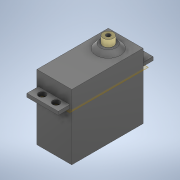
# Autodesk Inventor part: HX-15CS_15KGs_metal_gear_servo
Saved by Autodesk Inventor 2020 (Build 240168000, 168)
## iProperties
Created: 2019-12-03
Part Number: HX-15CS_15KGs_metal_gear_servo
Material: Generic
Document SubType Name: Modeling
Designer: maste
Density: 1 g/cm^3
Appearance: Smooth - Black
Author: maste
Autodesk Inventor part; units mm, degrees
ref_plane "YZ Plane" through (0, 0, 0) normal (1, 0, 0) x (0, 1, 0)
ref_plane "XY Plane" through (0, 0, 0) normal (0, 0, 1) x (1, 0, 0)
sketch "Sketch1" plane through (0, 0, 0) normal (0, 1, 0) x (-1, 0, 0)
  line L0 (20, 0) -> (0, 0)
  line L1 (0, 0) -> (0, -41)
  line L2 (0, -41) -> (20, -41)
  line L3 (20, -41) -> (20, 0)
  dimension "d0" = 20
  dimension "d1" = 41
  constraints: 8 end point, 2 parallel, 1 coincident, 1 horizontal, 1 perpendicular
  measures "d0" distance of L0.start L0.end
  measures "d1" distance of L0.end L1.end
extrude "Extrusion1" add sketch "Sketch1" along normal blind 37.5
sketch "Sketch2" plane through (0, 37.5, 0) normal (0, 1, 0) x (1, 0, 0)
  circle A0 centre (-10, 31) radius 3
  line L0 (-20, 41) -> (-20, 0) projected
  line L1 (0, 41) -> (-20, 41) projected
  point P0 (0, 0)
  dimension "d4" = 6
  dimension "d5" = 10
  dimension "d6" = 10
  constraints: 1 centre point
  measures "d4" diameter of A0
  measures "d5" distance from line of L0 A0.centre
  measures "d6" distance from line of L1 A0.centre
extrude "Extrusion2" add sketch "Sketch2" along normal blind 6.5
sketch "Sketch3" plane through (0, 37.5, 0) normal (0, 1, 0) x (1, 0, 0)
  circle A0 centre (-10, 31) radius 3 projected
  circle A1 centre (-10, 31) radius 7
  point P0 (0, 0)
  dimension "d9" = 14
  constraints: 1 centre point, 1 coincident
  measures "d9" diameter of A1
extrude "Extrusion3" add sketch "Sketch3" along normal blind 2.5
chamfer "Chamfer1" distance 2.5 angle 45 1 edges at (-17, 40, -31)
ref_plane "Work Plane1" through (0, 27.5, 0) normal (0, 1, 0) x (-1, 0, 0)
sketch "Sketch4" plane through (0, 27.5, 0) normal (0, 1, 0) x (-1, 0, 0)
  line L0 (19, -47.75) -> (1, -47.75)
  line L1 (1, -47.75) -> (1, 6.75)
  line L2 (1, 6.75) -> (19, 6.75)
  line L3 (19, 6.75) -> (19, -47.75)
  line L4 (0, 0) -> (0, -41) projected
  line L5 (0, -41) -> (20, -41) projected
  line L6 (14, -44) -> (6, -44) construction
  line L7 (6, -44) -> (6, 3) construction
  line L8 (6, 3) -> (14, 3) construction
  line L9 (14, 3) -> (14, -44) construction
  circle A0 centre (14, -44) radius 2
  circle A1 centre (6, -44) radius 2
  circle A2 centre (14, 3) radius 2
  circle A3 centre (6, 3) radius 2
  dimension "d16" = 54.5
  dimension "d17" = 18
  dimension "d18" = 1
  dimension "d19" = 6.75
  dimension "d20" = 47
  dimension "d21" = 8
  dimension "d22" = 5
  dimension "d23" = 3.75
  dimension "d24" = 4
  dimension "d25" = 4
  dimension "d26" = 4
  dimension "d27" = 4
  constraints: 16 end point, 4 centre point, 4 coincident, 4 parallel, 2 horizontal, 2 perpendicular
  measures "d16" distance of L0.end L1.end
  measures "d17" distance of L0.start L0.end
  measures "d18" distance between parallel lines of L4 L1
  measures "d19" distance between parallel lines of L5 L0
  measures "d20" distance of L6.end L7.end
  measures "d21" distance of L6.start L6.end
  measures "d22" distance between parallel lines of L3 L9
  measures "d23" distance between parallel lines of L2 L8
  measures "d24" diameter of A0
  measures "d25" diameter of A1
  measures "d26" diameter of A2
  measures "d27" diameter of A3
extrude "Extrusion4" add sketch "Sketch4" along normal blind 2
sketch "Sketch5" plane through (-10, 44, -31) normal (0, 1, 0) x (1, 0, 0)
  circle A0 centre (0, 0) radius 3 projected
  circle A1 centre (0, 0) radius 1.25
  point P0 (10, -31)
  dimension "d30" = 2.5
  constraints: 1 centre point, 1 coincident
  measures "d30" diameter of A1
extrude "Extrusion5" cut sketch "Sketch5" against normal blind 5 contours A1
sketch "Sketch6" plane through (0, 0, -41) normal (0, 0, -1) x (-1, 0, 0)
  line L0 (6.75, 9.5) -> (13.25, 9.5)
  line L1 (13.25, 9.5) -> (13.25, 5.5)
  line L2 (13.25, 5.5) -> (6.75, 5.5)
  line L3 (6.75, 5.5) -> (6.75, 9.5)
  line L4 (0, 0) -> (20, 0) projected
  line L5 (0, 0) -> (0, 37.5) projected
  dimension "d33" = 4
  dimension "d34" = 6.5
  dimension "d35" = 5.5
  dimension "d36" = 6.75
  constraints: 8 end point, 2 parallel, 1 horizontal, 1 perpendicular
  measures "d33" distance of L0.end L1.end
  measures "d34" distance of L0.start L0.end
  measures "d35" distance between parallel lines of L4 L2
  measures "d36" distance between parallel lines of L5 L3
extrude "Extrusion6" add sketch "Sketch6" along normal blind 4.5
draft "FaceDraft1" angle 2.5 pull direction (0, 0, -1) faces at (-6.75, 8.1667, -42.5) fixed edges at (-6.75, 7.5, -45.5)
draft "FaceDraft2" angle 2.5 pull direction (0, 0, -1) faces at (-8.8512, 5.5, -42.5) fixed edges at (-10, 5.5, -45.5)
draft "FaceDraft3" angle 2.5 pull direction (0, 0, -1) faces at (-8.8512, 9.5, -42.5) fixed edges at (-10, 9.5, -45.5)
draft "FaceDraft4" angle 2.5 pull direction (0, 0, -1) faces at (-13.25, 6.8333, -42.5) fixed edges at (-13.25, 7.5, -41)
body "Solid1"
